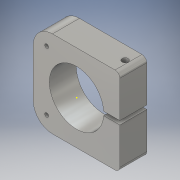
# Autodesk Inventor part: mOTORHOLDER
Saved by Autodesk Inventor 2016 (Build 200138000, 138)
## iProperties
Created: 2017-12-20
Part Number: mOTORHOLDER
Material: Generic
Document SubType Name: Modeling
Designer: student
Density: 1 g/cm^3
Appearance: Default
Author: student
Autodesk Inventor part; units mm, degrees
ref_plane "YZ Plane" through (0, 0, 0) normal (1, 0, 0) x (0, 1, 0)
ref_plane "XZ Plane" through (0, 0, 0) normal (0, 1, 0) x (-1, 0, 0)
ref_plane "XY Plane" through (0, 0, 0) normal (0, 0, 1) x (1, 0, 0)
sketch "Sketch1" plane through (0, 0, 0) normal (0, 0, 1) x (1, 0, 0)
  line L0 (-15.875, -28.575) -> (25.4, -28.575)
  line L1 (25.4, 28.575) -> (-15.875, 28.575)
  line L2 (-28.575, 15.875) -> (-28.575, -15.875)
  line L3 (-28.575, -28.575) -> (28.575, 28.575) construction
  line L4 (28.575, -28.575) -> (-28.575, 28.575) construction
  arc A0 (-15.875, 28.575) -> (-28.575, 15.875) centre (-15.875, 15.875) ccw
  arc A1 (-28.575, -15.875) -> (-15.875, -28.575) centre (-15.875, -15.875) ccw
  arc A2 (28.575, 25.4) -> (25.4, 28.575) centre (25.4, 25.4) ccw
  arc A3 (25.4, -28.575) -> (28.575, -25.4) centre (25.4, -25.4) ccw
  arc A4 (17.9256, 1.27) -> (17.9256, -1.27) centre (0, 0) ccw
  line L5 (18.2118, 5.08) -> (18.2118, -5.08) construction
  line L6 (17.9256, 1.27) -> (28.575, 1.27)
  line L7 (17.9256, -1.27) -> (28.575, -1.27)
  line L8 (28.575, -25.4) -> (28.575, -1.27)
  line L9 (28.575, 1.27) -> (28.575, 25.4)
  point P0 (23.2503, 1.27)
  point P1 (23.2503, -1.27)
  dimension "d0" = 57.15
  dimension "d1" = 57.15
  dimension "d2" = 12.7
  dimension "d3" = 3.175
  dimension "d5" = 10.16
  dimension "d8" = 28.575
  dimension "d11" = 57.15
  dimension "d14" = 2.54
  dimension "d23" = 35.941
  constraints: 20 end point, 10 point on circle, 10 tangent, 6 perpendicular, 6 point on line, 5 centre point, 4 midpoint, 3 parallel, 2 equal radius, 1 coincident, 1 horizontal, 1 vertical, 1 vertical alignment
  measures "d0" distance of L3.end L4.end
  measures "d1" distance of L4.start L3.end
  measures "d2" radius of A0
  measures "d3" radius of A2
  measures "d5" distance of L5.start L5.end
  measures "d8" distance from line of point (0, 0) L0
  measures "d11" distance between parallel lines of L2 L8
  measures "d14" distance between parallel lines of L7 L6
  measures "d23" diameter of A4
extrude "Extrusion1" add sketch "Sketch1" along normal blind 17.78
sketch "Sketch2" plane through (17.9256, -1.27, 0) normal (0, 1, 0) x (1, 0, 0)
  line L0 (0, 0) -> (10.6494, 0) projected
  line L1 (0, 0) -> (0, -17.78) projected
  line L2 (10.6494, -17.78) -> (0, -17.78) projected
  line L3 (10.6494, 0) -> (10.6494, -17.78) projected
  circle A0 centre (5.2706, -8.89) radius 1.27
  point P0 (-17.9256, 0)
  dimension "d15" = 2.54
  constraints: 1 centre point
  measures "d15" diameter of A0
hole "Hole1" at (23.1962, -1.27, 8.89) direction (0, -1, 0) diameter 2.54 end through all
sketch "Sketch3" plane through (-15.875, -28.575, 0) normal (0, -1, 0) x (1, 0, 0)
  circle A0 centre (39.0712, 8.89) radius 1.27 projected
  point P0 (15.875, 0)
  point P1 (38.1, 9.7084)
  point P2 (38.1, 8.0716)
  constraints: 1 vertical alignment
hole "Hole2" at (23.1962, -28.575, 8.89) direction (0, 1, 0) diameter 4.064 end through all counterbore diameter 7.62 counterbore depth 6.35
sketch "Sketch4" plane through (0, 0, 17.78) normal (0, 0, 1) x (1, 0, 0)
  point P0 (0, 0)
sketch "Sketch5" plane through (0, 0, 17.78) normal (0, 0, 1) x (1, 0, 0)
  point P0 (0, 0)
sketch "Sketch6" plane through (0, 0, 17.78) normal (0, 0, 1) x (1, 0, 0)
  line L0 (25.4, 28.575) -> (-15.875, 28.575) projected
  arc A0 (-15.875, 28.575) -> (-28.575, 15.875) centre (-15.875, 15.875) ccw projected
  line L1 (-28.575, 15.875) -> (-28.575, -15.875) projected
  arc A1 (-28.575, -15.875) -> (-15.875, -28.575) centre (-15.875, -15.875) ccw projected
  line L2 (-15.875, -28.575) -> (25.4, -28.575) projected
  arc A2 (25.4, -28.575) -> (28.575, -25.4) centre (25.4, -25.4) ccw projected
  line L3 (28.575, -25.4) -> (28.575, -1.27) projected
  line L4 (28.575, -1.27) -> (17.9256, -1.27) projected
  arc A3 (17.9256, 1.27) -> (17.9256, -1.27) centre (0, 0) ccw projected
  line L5 (17.9256, 1.27) -> (28.575, 1.27) projected
  line L6 (28.575, 1.27) -> (28.575, 25.4) projected
  arc A4 (28.575, 25.4) -> (25.4, 28.575) centre (25.4, 25.4) ccw projected
  circle A5 centre (-19.685, -19.685) radius 1.27
  circle A6 centre (-19.685, 19.685) radius 1.27
  dimension "d31" = 2.54
  dimension "d32" = 3.81
  dimension "d33" = 3.81
  dimension "d34" = 2.54
  dimension "d35" = 3.81
  dimension "d36" = 3.81
  constraints: 2 centre point
  measures "d31" diameter of A5
  measures "d32" horizontal distance of A1.centre A5.centre
  measures "d33" horizontal distance of A1.centre A5.centre
  measures "d34" diameter of A6
  measures "d35" horizontal distance of A0.centre A6.centre
  measures "d36" horizontal distance of A0.centre A6.centre
extrude "Extrusion2" cut sketch "Sketch6" against normal blind 25.4 contours A5 | A6
body "Solid1"
